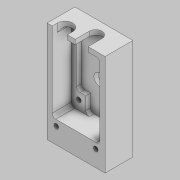
# Autodesk Inventor part: case
Saved by Autodesk Inventor 2021.4 (Build 254397000, 397)
## iProperties
Created: 2022-10-31
Part Number: case
Material: Generisch
Document SubType Name: Modeling
Designer: Tilman Preuschoff
Density: 1 g/cm^3
Appearance: Vorgabe
Author: Tilman Preuschoff
Autodesk Inventor part; units mm, degrees
ref_plane "YZ Plane" through (0, 0, 0) normal (1, 0, 0) x (0, 1, 0)
ref_plane "XZ Plane" through (0, 0, 0) normal (0, 1, 0) x (-1, 0, 0)
ref_plane "XY Plane" through (0, 0, 0) normal (0, 0, 1) x (1, 0, 0)
sketch "Skizze1" plane through (0, 0, 0) normal (0, 0, 1) x (1, 0, 0)
  line L0 (-12.5, 21.75) -> (12.5, 21.75)
  line L1 (12.5, 21.75) -> (12.5, -21.75)
  line L2 (12.5, -21.75) -> (-12.5, -21.75)
  line L3 (-12.5, -21.75) -> (-12.5, 21.75)
  line L4 (-12.5, 21.75) -> (12.5, -21.75) construction
  line L5 (12.5, 21.75) -> (-12.5, -21.75) construction
  point P0 (0, 0)
  dimension "d0" = 25
  dimension "d1" = 43.5
  constraints: 12 end point, 2 midpoint, 2 parallel, 1 horizontal, 1 perpendicular
  measures "d0" distance between parallel lines of L1 L3
  measures "d1" distance between parallel lines of L0 L2
extrude "Extrusion1" add sketch "Skizze1" along normal blind 12
sketch "Skizze2" plane through (0, 0, 12) normal (0, 0, 1) x (1, 0, 0)
  line L0 (-8.75, 19.75) -> (8.75, 19.75)
  line L1 (10.25, 18.25) -> (10.25, -10.75)
  line L2 (8.75, -12.25) -> (-8.75, -12.25)
  line L3 (-10.25, -10.75) -> (-10.25, 18.25)
  line L4 (-10.25, 19.75) -> (10.25, -12.25) construction
  line L5 (10.25, 19.75) -> (-10.25, -12.25) construction
  line L6 (12.5, 21.75) -> (-12.5, 21.75) projected
  arc A0 (-8.75, 19.75) -> (-10.25, 18.25) centre (-8.75, 18.25) ccw
  arc A1 (10.25, 18.25) -> (8.75, 19.75) centre (8.75, 18.25) ccw
  arc A2 (8.75, -12.25) -> (10.25, -10.75) centre (8.75, -10.75) ccw
  arc A3 (-10.25, -10.75) -> (-8.75, -12.25) centre (-8.75, -10.75) ccw
  point P0 (0, 0)
  point P1 (0, 3.75)
  point P2 (0, 3.75)
  dimension "d4" = 20.5
  dimension "d5" = 2
  dimension "d6" = 32
  dimension "d7" = 1.5
  constraints: 12 end point, 8 point on circle, 8 point on line, 8 tangent, 4 centre point, 3 equal radius, 3 midpoint, 2 parallel, 1 horizontal, 1 perpendicular, 1 vertical alignment
  measures "d4" distance between parallel lines of L1 L3
  measures "d5" distance between parallel lines of L6 L0
  measures "d6" distance between parallel lines of L2 L0
  measures "d7" radius of A0
extrude "Extrusion2" cut sketch "Skizze2" against normal blind 8.2
sketch "Skizze3" plane through (0, 0, 3.8) normal (0, 0, 1) x (1, 0, 0)
  line L0 (-7, -8.25) -> (7, -8.25)
  line L1 (-8.75, 19.75) -> (8.75, 19.75) projected
  point P0 (0, 0)
  dimension "d10" = 14
  dimension "d11" = 7
  dimension "d12" = 28
  constraints: 2 end point, 1 horizontal
  measures "d10" distance of L0.end L0.start
  measures "d11" horizontal distance of L0.end point (0, 0)
  measures "d12" distance between parallel lines of L0 L1
hole "Bohrung1" at (-7, -8.25, 3.8) at (7, -8.25, 3.8) direction (0, 0, -1) diameter 2.013 end through all thread size "M2.5x0.45" class "6H" standard "ISO Metric profile"
sketch "Skizze4" plane through (0, 0, 3.8) normal (0, 0, 1) x (1, 0, 0)
  circle A0 centre (7, -8.25) radius 1.0065 projected
  point P0 (0, 0)
  point P1 (0, 1.75)
  dimension "d20" = 10
  constraints: 1 vertical alignment
  measures "d20" vertical distance of A0.centre point (0, 1.75)
hole "Bohrung2" at (0, 1.75, 3.8) direction (0, 0, -1) diameter 5 end through all
sketch "Skizze5" plane through (0, 0, 3.8) normal (0, 0, 1) x (1, 0, 0)
  line L0 (-8.75, 19.75) -> (8.75, 19.75) projected
  line L1 (-6.45, 19.75) -> (6.95, 19.75)
  line L2 (7.95, 21) -> (7.95, 13.25)
  line L3 (6.45, 11.75) -> (-6.45, 11.75)
  line L4 (-7.95, 13.25) -> (-7.95, 18.25)
  arc A0 (-6.45, 19.75) -> (-7.95, 18.25) centre (-6.45, 18.25) ccw
  arc A1 (6.45, 11.75) -> (7.95, 13.25) centre (6.45, 13.25) ccw
  arc A2 (-7.95, 13.25) -> (-6.45, 11.75) centre (-6.45, 13.25) ccw
  line L5 (10.25, 18.25) -> (10.25, -10.75) projected
  line L6 (6.95, 19.75) -> (6.45, 19.75)
  line L7 (7.95, 21) -> (7.95, 18.25)
  arc A3 (7.95, 18.25) -> (6.45, 19.75) centre (6.45, 18.25) ccw
  line L8 (-10.25, -10.75) -> (-10.25, 18.25) projected
  line L9 (-7.95, 13.25) -> (7.95, 13.25)
  line L10 (7.95, 13.25) -> (7.95, -3.75)
  line L11 (6.45, -5.25) -> (-6.45, -5.25)
  line L12 (-7.95, -3.75) -> (-7.95, 13.25)
  arc A4 (-7.95, -3.75) -> (-6.45, -5.25) centre (-6.45, -3.75) ccw
  arc A5 (6.45, -5.25) -> (7.95, -3.75) centre (6.45, -3.75) ccw
  circle A6 centre (7, -8.25) radius 1.0065 projected
  line L13 (8.75, -12.25) -> (-8.75, -12.25) projected
  line L14 (-4, -5.25) -> (4, -5.25)
  line L15 (4, -5.25) -> (4, -10.75)
  line L16 (2.5, -12.25) -> (-2.5, -12.25)
  line L17 (-4, -10.75) -> (-4, -5.25)
  circle A7 centre (-7, -8.25) radius 1.0065 projected
  arc A8 (-4, -10.75) -> (-2.5, -12.25) centre (-2.5, -10.75) ccw
  arc A9 (2.5, -12.25) -> (4, -10.75) centre (2.5, -10.75) ccw
  point P0 (0, 0)
  point P1 (-7.95, 19.75)
  point P2 (7.95, 19.75)
  point P3 (7.95, 18.25)
  point P4 (4, -12.25)
  point P5 (4, -5.25)
  dimension "d28" = 1.5
  dimension "d29" = 2.3
  dimension "d31" = 8
  dimension "d39" = 1.5
  dimension "d67" = 1.5
  dimension "d73" = 2.3
  dimension "d74" = 1.5
  dimension "d75" = 3
  dimension "d76" = 3
  dimension "d77" = 3
  dimension "d78" = 1.5
  constraints: 28 end point, 16 point on circle, 16 tangent, 10 point on line, 8 centre point, 6 parallel, 4 perpendicular, 3 equal radius, 3 horizontal, 1 vertical alignment
  measures "d28" radius of A0
  measures "d29" distance between parallel lines of L5 L2
  measures "d31" distance between parallel lines of L3 L0
  measures "d39" radius of A3
  measures "d67" radius of A1
  measures "d73" distance between parallel lines of L8 L4
  measures "d74" radius of A4
  measures "d75" distance from line of A6.centre L11
  measures "d76" distance from line of A6.centre L15
  measures "d77" distance from line of A7.centre L17
  measures "d78" radius of A8
sketch "Skizze6" plane through (0, 0, 12) normal (0, 0, 1) x (1, 0, 0)
  line L0 (12.5, 21.75) -> (-12.5, 21.75) projected
  line L1 (-8.75, 19.75) -> (8.75, 19.75) projected
  line L2 (-1.1, 21.75) -> (5.9, 21.75)
  line L3 (5.9, 21.75) -> (5.9, 19.75)
  line L4 (5.9, 19.75) -> (-1.1, 19.75)
  line L5 (-1.1, 19.75) -> (-1.1, 21.75)
  line L6 (12.5, -21.75) -> (12.5, 21.75) projected
  line L7 (7.95, 22) -> (7.95, 17) projected
  point P0 (0, 0)
  point P1 (6.95, 22)
  point P2 (5.9, 20.75)
  point P3 (7.95, 19.5)
  dimension "d34" = 7
  dimension "d38" = 6.6
  constraints: 8 end point, 2 midpoint, 2 parallel, 1 horizontal, 1 perpendicular, 1 point on line, 2 other
  measures "d34" distance between parallel lines of L3 L5
  measures "d38" distance between parallel lines of L6 L3
extrude "Extrusion4" [suppressed]
extrude "Extrusion5" cut sketch "Skizze5" against normal blind 2 contours L0 A3 L2 L9 L4 A0 | L9 A1 L3 A2 | A2 L3 A1 L10 A5 L11 A4 L12 | L11 L15 A9 L13 A8 L17
sketch "Skizze7" plane through (-12.5, -21.75, 0) normal (0, -1, 0) x (1, 0, 0)
  line L0 (0, 0) -> (25, 0) projected
  point P0 (12.5, 0)
  point P1 (12.5, 7)
  point P2 (12.5, 0)
  dimension "d42" = 7
  constraints: 1 midpoint, 1 vertical alignment
  measures "d42" distance from line of point (12.5, 7) L0
hole "Bohrung3" at (0, -21.75, 7) direction (0, 1, 0) diameter 4.917 depth 7 tip angle 118 thread size "M6x1" class "6H" standard "ISO Metric profile"
sketch "Skizze8" plane through (0, 0, 12) normal (0, 0, 1) x (1, 0, 0)
  line L0 (-12.5, -21.75) -> (12.5, -21.75) projected
  line L1 (-12.5, 21.75) -> (-12.5, -21.75) projected
  line L2 (12.5, -21.75) -> (12.5, 21.75) projected
  point P0 (0, 0)
  point P1 (-8.5, -14.75)
  point P2 (8.5, -14.75)
  dimension "d50" = 7
  dimension "d51" = 4
  dimension "d52" = 4
  constraints: 1 horizontal alignment
  measures "d50" distance from line of L0 point (-8.5, -14.75)
  measures "d51" distance from line of L1 point (-8.5, -14.75)
  measures "d52" distance from line of L2 point (8.5, -14.75)
hole "Bohrung4" at (-8.5, -14.75, 12) at (8.5, -14.75, 12) direction (0, 0, -1) diameter 2.013 depth 8 tip angle 118 thread size "M2.5x0.45" class "6H" standard "ISO Metric profile"
sketch "Skizze10" plane through (-12.5, 21.75, 0) normal (0, 1, 0) x (1, 0, 0)
  line L0 (2.25, -12) -> (8.75, -12)
  line L1 (8.75, -12) -> (8.75, -9.75)
  line L2 (8.75, -9.75) -> (2.25, -9.75)
  line L3 (2.25, -9.75) -> (2.25, -12)
  circle A0 centre (5.5, -9.75) radius 3.25
  point P0 (12.5, 0)
  point P1 (2.25, -9.75)
  dimension "d63" = 6.5
  dimension "d64" = 2.25
  constraints: 8 end point, 2 parallel, 1 horizontal, 1 midpoint, 1 perpendicular, 3 other
  measures "d63" distance between parallel lines of L1 L3
  measures "d64" distance from line of point (5.5, -9.75) L0
extrude "Extrusion7" cut sketch "Skizze10" against normal blind 10 contours L3 A0 L0 | A0 L2 L0 | A0 L2 | A0 L1 L0
sketch "Skizze11" plane through (-12.5, 21.75, 0) normal (0, 1, 0) x (1, 0, 0)
  line L0 (8.75, -12) -> (21.25, -12) projected
  line L1 (12.15, -12) -> (17.65, -12)
  line L2 (17.65, -12) -> (17.65, -6)
  line L3 (17.65, -6) -> (12.15, -6)
  line L4 (12.15, -6) -> (12.15, -12)
  line L5 (25, 0) -> (25, -12) projected
  circle A0 centre (14.9, -6) radius 2.75
  point P0 (12.5, 0)
  dimension "d68" = 5.5
  dimension "d69" = 7.35
  dimension "d70" = 6
  constraints: 8 end point, 2 parallel, 1 horizontal, 1 midpoint, 1 perpendicular, 1 point on line, 3 other
  measures "d68" distance between parallel lines of L2 L4
  measures "d69" distance between parallel lines of L5 L2
  measures "d70" distance between parallel lines of L0 L3
extrude "Extrusion8" cut sketch "Skizze11" against normal up to surface (2 mm away)
